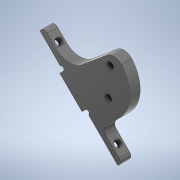
# Autodesk Inventor part: Camera_vertical_frame_01
Saved by Autodesk Inventor 2020.4 (Build 244396010, 396A)
## iProperties
Created: 2021-09-12
Part Number: Camera_vertical_frame_01
Material: CFRP
Document SubType Name: Modeling
Designer: t-nagamine
Density: 1.43 g/cm^3
Appearance: 滑らか - 黒
Author: t-nagamine
Autodesk Inventor part; units mm, degrees
ref_plane "YZ Plane" through (0, 0, 0) normal (1, 0, 0) x (0, 1, 0)
ref_plane "XZ Plane" through (0, 0, 0) normal (0, 1, 0) x (-1, 0, 0)
ref_plane "XY Plane" through (0, 0, 0) normal (0, 0, 1) x (1, 0, 0)
derived "Head_vertical_frame_01.ipt"
sketch "スケッチ1" plane through (0, 0, 0) normal (0, 0, 1) x (1, 0, 0)
  line L0 (0, 0) -> (27, 0) construction
  line L1 (27, 0) -> (27, 5) construction
  line L2 (27, 5) -> (0, 5) construction
  line L3 (0, 5) -> (0, 0) construction
  line L4 (0, 2.5) -> (27, 2.5) construction
  line L5 (13.5, 5) -> (13.5, 0) construction
  circle A0 centre (3.7, 2.5) radius 1.55
  line L6 (7.5, 5) -> (7.5, 0) construction
  line L7 (19.5, 5) -> (19.5, 0) construction
  circle A1 centre (23.3, 2.5) radius 1.55
  line L8 (7.49, 5.01) -> (9.59, 5.01) construction
  line L9 (19.51, 5.01) -> (19.51, -0.01)
  line L10 (19.51, -0.01) -> (7.49, -0.01)
  line L11 (7.49, -0.01) -> (7.49, 5.01)
  line L12 (7.49, 5.01) -> (19.51, -0.01) construction
  line L13 (19.51, 5.01) -> (7.49, -0.01) construction
  line L14 (0, 0) -> (7.5, -2)
  line L15 (7.5, -2) -> (19.5, -2)
  line L16 (27, 0) -> (19.5, -2)
  arc A2 (9.59, 5.01) -> (7.49, 5.01) centre (8.54, 5.01) ccw
  arc A3 (19.51, 5.01) -> (17.41, 5.01) centre (18.46, 5.01) ccw
  line L17 (9.59, 5.01) -> (17.41, 5.01)
  line L18 (9.59, -0.01) -> (7.49, -0.01)
  line L19 (17.41, 5.01) -> (19.51, 5.01) construction
  line L20 (27, 7) -> (0, 7) construction
  line L21 (0, 0) -> (0, 7)
  line L22 (12.1912, 40) -> (12.1912, 35) construction
  circle A4 centre (14.8912, 37.5) radius 1.55
  line L23 (37.1912, 35) -> (37.1912, 40) construction
  line L24 (30.6912, 40) -> (30.6912, 35) construction
  circle A5 centre (34.4912, 37.5) radius 1.55
  line L25 (30.7012, 40.01) -> (30.7012, 34.99)
  line L26 (18.6912, 40) -> (18.6912, 35) construction
  line L27 (12.1912, 35) -> (37.1912, 35) construction
  line L28 (37.1912, 40) -> (12.1912, 40) construction
  line L29 (12.1912, 37.5) -> (37.1912, 37.5) construction
  line L30 (24.6912, 40) -> (24.6912, 35) construction
  line L31 (20.7812, 40.01) -> (28.6012, 40.01)
  line L32 (28.6012, 34.99) -> (20.7812, 34.99)
  line L33 (18.6812, 40.01) -> (30.7012, 34.99) construction
  line L34 (30.7012, 40.01) -> (18.6812, 34.99) construction
  arc A6 (30.7012, 40.01) -> (28.6012, 40.01) centre (29.6512, 40.01) ccw
  line L35 (28.6012, 40.01) -> (30.7012, 40.01) construction
  arc A7 (28.6012, 34.99) -> (30.7012, 34.99) centre (29.6512, 34.99) ccw
  line L36 (30.7012, 34.99) -> (28.6012, 34.99) construction
  line L37 (18.6812, 40.01) -> (20.7812, 40.01) construction
  line L38 (20.7812, 34.99) -> (18.6812, 34.99) construction
  arc A8 (20.7812, 40.01) -> (18.6812, 40.01) centre (19.7312, 40.01) ccw
  arc A9 (18.6812, 34.99) -> (20.7812, 34.99) centre (19.7312, 34.99) ccw
  line L39 (18.6812, 34.99) -> (18.6812, 40.01)
  line L40 (18.6912, 73) -> (18.6912, 68) construction
  line L41 (18.6812, 67.99) -> (18.6812, 73.01)
  line L42 (20.7812, 67.99) -> (18.6812, 67.99) construction
  arc A10 (18.6812, 67.99) -> (20.7812, 67.99) centre (19.7312, 67.99) ccw
  arc A11 (20.7812, 73.01) -> (18.6812, 73.01) centre (19.7312, 73.01) ccw
  line L43 (24.6912, 73) -> (24.6912, 68) construction
  line L44 (12.1912, 70.5) -> (37.1912, 70.5) construction
  line L45 (37.1912, 73) -> (12.1912, 73) construction
  line L46 (12.1912, 68) -> (37.1912, 68) construction
  line L47 (30.7012, 73.01) -> (18.6812, 67.99) construction
  line L48 (18.6812, 73.01) -> (30.7012, 67.99) construction
  line L49 (28.6012, 67.99) -> (20.7812, 67.99)
  line L50 (20.7812, 73.01) -> (28.6012, 73.01)
  line L51 (37.1912, 68) -> (37.1912, 73) construction
  line L52 (18.6812, 73.01) -> (20.7812, 73.01) construction
  line L53 (30.6912, 73) -> (30.6912, 68) construction
  arc A12 (30.7012, 73.01) -> (28.6012, 73.01) centre (29.6512, 73.01) ccw
  line L54 (28.6012, 73.01) -> (30.7012, 73.01) construction
  line L55 (30.7012, 73.01) -> (30.7012, 67.99)
  line L56 (30.7012, 67.99) -> (28.6012, 67.99) construction
  circle A13 centre (34.4912, 70.5) radius 1.55
  arc A14 (28.6012, 67.99) -> (30.7012, 67.99) centre (29.6512, 67.99) ccw
  circle A15 centre (14.8912, 70.5) radius 1.55
  line L57 (12.1912, 73) -> (12.1912, 68) construction
  line L58 (27, 0) -> (27, 6.6473)
  line L59 (37.1912, 35) -> (27.1206, 7.3314)
  line L60 (11.8992, 39.6929) -> (0, 7)
  line L61 (37.1912, 35) -> (37.1912, 73)
  line L62 (6.8054, 101.4338) -> (6.7491, 101.3865)
  arc A16 (4.7394, 86.3065) -> (5.3203, 95.7003) centre (-4.8938, 91.617) ccw
  circle A17 centre (-4.8938, 91.617) radius 14.6063 construction
  line L63 (1.0459, 61.9185) -> (-21.5815, 84.5459) construction
  line L64 (-21.5815, 84.5459) -> (-18.0459, 88.0815) construction
  line L65 (-18.0459, 88.0815) -> (4.5815, 65.4541) construction
  line L66 (4.5815, 65.4541) -> (1.0459, 61.9185) construction
  line L67 (1.0459, 61.9185) -> (-18.0459, 88.0815) construction
  line L68 (-21.5815, 84.5459) -> (4.5815, 65.4541) construction
  line L69 (13.8495, 100.8175) -> (37.1912, 73)
  arc A18 (11.8992, 39.6929) -> (5.2055, 80.7796) centre (-28.1256, 54.2607) ccw
  arc A19 (8.344, 97.7899) -> (6.2953, 101.0057) centre (-4.8938, 91.617) ccw construction
  arc A20 (5.0756, 80.942) -> (7.4988, 83.886) centre (-4.8938, 91.617) ccw construction
  circle A21 centre (8.344, 97.7899) radius 1.65
  circle A22 centre (7.4988, 83.886) radius 1.65
  arc A23 (13.8495, 100.8175) -> (6.8054, 101.4338) centre (10.0193, 97.6035) ccw
  arc A24 (6.7491, 101.3865) -> (5.3203, 95.7003) centre (9.9631, 97.5563) ccw
  arc A25 (4.7394, 86.3065) -> (5.2055, 80.7796) centre (9.1182, 83.8926) ccw
  arc A26 (27.1206, 7.3314) -> (27, 6.6473) centre (29, 6.6473) ccw
  arc A27 (7.49, 1.4749) -> (8.9749, -0.01) centre (8.2325, 0.7325) ccw
  arc A28 (18.0251, -0.01) -> (19.51, 1.4749) centre (18.7675, 0.7325) ccw
  point P0 (13.5, 2.5)
  point P1 (24.6912, 37.5)
  point P2 (24.6912, 70.5)
  point P3 (10.6356, 104.6477)
  point P4 (3.5327, 98.6877)
  point P5 (-8.5, 75)
sketch "スケッチ2" plane through (0, 0, 0) normal (0, 0, 1) x (1, 0, 0)
  line L0 (-18.0459, 88.0815) -> (4.5815, 65.4541) construction
  line L1 (12.0061, 58.0294) -> (12.7132, 58.7365)
  line L2 (4.5815, 65.4541) -> (1.0459, 61.9185) construction
  line L3 (-25.4706, 95.5061) -> (-24.7635, 96.2132)
  line L4 (-21.5815, 84.5459) -> (-18.0459, 88.0815) construction
  line L5 (1.0459, 61.9185) -> (-21.5815, 84.5459) construction
  line L6 (-14.1851, 84.2207) -> (-15.8822, 82.5236)
  line L7 (-3.522, 73.5575) -> (-5.219, 71.8604)
  line L8 (-25.4706, 95.5061) -> (-15.6701, 85.7056)
  line L9 (-2.037, 72.0726) -> (12.0061, 58.0294)
  line L10 (-5.219, 71.8604) -> (-15.8822, 82.5236)
  arc A0 (-14.1851, 84.2207) -> (-15.6701, 85.7056) centre (-14.9276, 84.9631) ccw
  arc A1 (-2.037, 72.0726) -> (-3.522, 73.5575) centre (-2.7795, 72.815) ccw
  arc A2 (12.7132, 58.7365) -> (12.7132, 61.565) centre (11.299, 60.1508) ccw
  line L11 (12.7132, 61.565) -> (6.3492, 67.9289)
  arc A3 (6.3492, 71.7917) -> (6.3492, 67.9289) centre (8.2806, 69.8603) ccw
  arc A4 (-17.7629, 92.0413) -> (-5.0496, 91.4862) centre (-11.1034, 98.7008) ccw
  line L12 (-17.7629, 92.0413) -> (-21.9348, 96.2132)
  line L13 (-5.0496, 91.4862) -> (6.8054, 101.4338)
  arc A5 (13.8495, 100.8175) -> (6.8054, 101.4338) centre (10.0193, 97.6035) ccw
  arc A6 (12.8668, 78.3093) -> (13.8495, 100.8175) centre (1.0765, 90.0996) ccw
  line L14 (12.8668, 78.3093) -> (6.3492, 71.7917)
  arc A7 (-21.9348, 96.2132) -> (-24.7635, 96.2132) centre (-23.3491, 94.7989) ccw
  circle A8 centre (7.4988, 83.886) radius 1.65 projected
  circle A9 centre (8.344, 97.7899) radius 1.65 projected
  point P0 (0, 0)
  dimension "d3" = 1
  dimension "d4" = 0
  dimension "d5" = 10.5
  dimension "d6" = 1
  dimension "d7" = 0
  dimension "d8" = 53
  dimension "d9" = 2.4
  dimension "d10" = 15.96
  dimension "d11" = 2.4
  dimension "d12" = 21.96
  dimension "d14" = 2.1
  dimension "d15" = 2.1
  dimension "d17" = 1
  dimension "d18" = 2
  dimension "d22" = 9
  dimension "d23" = 3
  dimension "d25" = 2.7314
  dimension "d27" = 9.4179
  dimension "d28" = 5.9
  dimension "d29" = 5
  dimension "d30" = 6.5176
  constraints: 22 end point, 16 point on circle, 11 tangent, 8 centre point, 6 perpendicular, 2 line through centre, 2 parallel
  measures "d3" distance of L1.start L1.end
  measures "d4" distance from line of L0 L1.start
  measures "d5" distance between parallel lines of L2 L1
  measures "d6" distance of L3.end L3.start
  measures "d7" distance from line of L3.start L0
  measures "d8" distance between parallel lines of L3 L1
  measures "d9" distance of L6.start L6.end
  measures "d10" distance between parallel lines of L6 L3
  measures "d11" distance of L7.start L7.end
  measures "d12" distance between parallel lines of L1 L7
  measures "d14" distance of L8.end L6.start
  measures "d15" distance of L9.start L7.start
  measures "d17" distance from line of L9 A2.centre
  measures "d18" radius of A2
  measures "d22" distance of L11.start L11.end
  measures "d23" distance between parallel lines of L9 L11
  measures "d25" radius of A3
  measures "d27" radius of A4
  measures "d28" distance of L12.start L12.end
  measures "d29" radius of A5
  measures "d30" horizontal distance of L14.start L14.end
extrude "押し出し1" add sketch "スケッチ2" against normal blind 5
sketch "スケッチ3" plane through (-17.7629, 92.0413, -5) normal (0.7071068, 0.7071068, 0) x (-0.7071068, 0.7071068, 0)
  circle A0 centre (1.4002, 2.5) radius 1.65
  circle A1 centre (-38.5998, 2.5) radius 1.65
  line L0 (5.9, 0) -> (0, 0) projected
  line L1 (-34.0998, 0) -> (-43.0998, 0) projected
  line L2 (7.9002, 5) -> (7.9002, 0) projected
  line L3 (-45.0998, 5) -> (-45.0998, 0) projected
  point P0 (-77.6432, 5)
  dimension "d33" = 3.3
  dimension "d34" = 3.3
  dimension "d35" = 2.5
  dimension "d36" = 2.5
  dimension "d37" = 6.5
  dimension "d38" = 6.5
  constraints: 2 centre point
  measures "d33" diameter of A0
  measures "d34" diameter of A1
  measures "d35" distance from line of L0 A0.centre
  measures "d36" distance from line of L1 A1.centre
  measures "d37" distance from line of L2 A0.centre
  measures "d38" distance from line of A1.centre L3
extrude "押し出し2" cut sketch "スケッチ3" against normal through all
